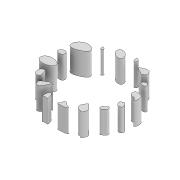
# Autodesk Inventor part: simple_ring3
Saved by Autodesk Inventor 2021 (Build 250183000, 183)
## iProperties
Created: 2022-04-12
Part Number: simple_ring3
Material: Generic
Document SubType Name: Modeling
Designer: Derm
Density: 1 g/cm^3
Appearance: Default
Author: Derm
Autodesk Inventor part; units mm, degrees
ref_plane "YZ Plane" through (0, 0, 0) normal (1, 0, 0) x (0, 1, 0)
ref_plane "XZ Plane" through (0, 0, 0) normal (0, 1, 0) x (-1, 0, 0)
ref_plane "XY Plane" through (0, 0, 0) normal (0, 0, 1) x (1, 0, 0)
sketch "Sketch1" plane through (0, 0, 0) normal (0, 1, 0) x (-1, 0, 0)
  line L0 (0, 0) -> (10000, 0)
  line L1 (0, 0) -> (9807.8528, -1950.9032) construction
  line L2 (-4839.2703, 7607.7402) -> (-4527.6462, 8434.2216) construction
  line L3 (-4527.6462, 8434.2216) -> (-5367.6765, 9477.4851) construction
  line L4 (-5367.6765, 9477.4851) -> (-6194.1579, 8840.6879) construction
  line L5 (-6194.1579, 8840.6879) -> (-6194.1579, 9938.1469) construction
  line L6 (-6194.1579, 9938.1469) -> (-6979.9927, 8718.748) construction
  line L7 (-6979.9927, 8718.748) -> (-7074.8348, 7865.1688) construction
  line L8 (-7074.8348, 7865.1688) -> (-6248.3534, 7350.3115) construction
  line L9 (-6248.3534, 7350.3115) -> (-5462.5186, 6158.0104) construction
  line L10 (-5462.5186, 6158.0104) -> (-5282.6353, 7062.3446) construction
  line L11 (-5282.6353, 7062.3446) -> (-4839.2703, 7607.7402) construction
  spline S0 degree 4 poles (-4839.2703, 7607.7402) (-4527.6462, 8434.2216) (-5367.6765, 9477.4851) (-6194.1579, 8840.6879) (-6194.1579, 9938.1469) (-6979.9927, 8718.748) (-7074.8348, 7865.1688) (-6248.3534, 7350.3115) (-5462.5186, 6158.0104) (-5282.6353, 7062.3446) (-4839.2703, 7607.7402) knots 1 1 1 1 1 2 3 4 5 6 7 8 8 8 8 8
  line L12 (-8998.7753, -2526.8192) -> (-8511.0158, -1632.5933) construction
  line L13 (-8511.0158, -1632.5933) -> (-9486.5348, -711.2697) construction
  line L14 (-9486.5348, -711.2697) -> (-10258.8207, -1293.8714) construction
  line L15 (-10258.8207, -1293.8714) -> (-10773.678, -386.0967) construction
  line L16 (-10773.678, -386.0967) -> (-10673.6173, 116.9424) construction
  line L17 (-10673.6173, 116.9424) -> (-11274.9864, -657.0742) construction
  line L18 (-11274.9864, -657.0742) -> (-11274.9864, -1402.2624) construction
  line L19 (-11274.9864, -1402.2624) -> (-10976.9111, -2526.8192) construction
  line L20 (-10976.9111, -2526.8192) -> (-9807.8528, -2526.8192) construction
  line L21 (-9807.8528, -2526.8192) -> (-8998.7753, -2526.8192) construction
  spline S1 degree 4 poles (-8998.7753, -2526.8192) (-8511.0158, -1632.5933) (-9486.5348, -711.2697) (-10258.8207, -1293.8714) (-10773.678, -386.0967) (-10673.6173, 116.9424) (-11274.9864, -657.0742) (-11274.9864, -1402.2624) (-10976.9111, -2526.8192) (-9807.8528, -2526.8192) (-8998.7753, -2526.8192) knots 1 1 1 1 1 2 3 4 5 6 7 8 8 8 8 8
  line L22 (-3999.2401, -8583.1668) -> (-3999.2401, -7924.4901) construction
  line L23 (-3999.2401, -7924.4901) -> (-5354.1276, -7924.4901) construction
  line L24 (-5354.1276, -7924.4901) -> (-5354.1276, -7119.8881) construction
  line L25 (-5354.1276, -7119.8881) -> (-6085.7669, -7445.0612) construction
  line L26 (-6085.7669, -7445.0612) -> (-7020.6393, -7924.4901) construction
  line L27 (-7020.6393, -7924.4901) -> (-6397.391, -8420.5803) construction
  line L28 (-6397.391, -8420.5803) -> (-6500.0442, -8936.6526) construction
  line L29 (-6500.0442, -8936.6526) -> (-5476.0675, -9436.746) construction
  line L30 (-5476.0675, -9436.746) -> (-4500.5485, -8799.9488) construction
  line L31 (-4500.5485, -8799.9488) -> (-3999.2401, -8583.1668) construction
  spline S2 degree 4 poles (-3999.2401, -8583.1668) (-3999.2401, -7924.4901) (-5354.1276, -7924.4901) (-5354.1276, -7119.8881) (-6085.7669, -7445.0612) (-7020.6393, -7924.4901) (-6397.391, -8420.5803) (-6500.0442, -8936.6526) (-5476.0675, -9436.746) (-4500.5485, -8799.9488) (-3999.2401, -8583.1668) knots 1 1 1 1 1 2 3 4 5 6 7 8 8 8 8 8
  line L32 (8005.0639, 4532.1453) -> (7747.6353, 4911.5139) construction
  line L33 (7747.6353, 4911.5139) -> (7747.6353, 5697.3487) construction
  line L34 (7747.6353, 5697.3487) -> (7232.778, 6103.815) construction
  line L35 (7232.778, 6103.815) -> (7476.6578, 6605.1234) construction
  line L36 (7476.6578, 6605.1234) -> (8314.6961, 7025.1386) construction
  line L37 (8314.6961, 7025.1386) -> (9075.4251, 6225.7549) construction
  line L38 (9075.4251, 6225.7549) -> (9075.4251, 5656.7021) construction
  line L39 (9075.4251, 5656.7021) -> (9075.4251, 5074.1004) construction
  line L40 (9075.4251, 5074.1004) -> (8723.1543, 4626.9875) construction
  line L41 (8723.1543, 4626.9875) -> (8005.0639, 4532.1453) construction
  spline S3 degree 4 poles (8005.0639, 4532.1453) (7747.6353, 4911.5139) (7747.6353, 5697.3487) (7232.778, 6103.815) (7476.6578, 6605.1234) (8314.6961, 7025.1386) (9075.4251, 6225.7549) (9075.4251, 5656.7021) (9075.4251, 5074.1004) (8723.1543, 4626.9875) (8005.0639, 4532.1453) knots 1 1 1 1 1 2 3 4 5 6 7 8 8 8 8 8
  line L42 (2531.318, 10954.3126) -> (2531.318, 10073.6357) construction
  line L43 (2531.318, 10073.6357) -> (2436.4759, 8786.4924) construction
  line L44 (2436.4759, 8786.4924) -> (1460.9569, 9260.7031) construction
  line L45 (1460.9569, 9260.7031) -> (1460.9569, 9965.2447) construction
  line L46 (1460.9569, 9965.2447) -> (878.3552, 10845.9216) construction
  line L47 (878.3552, 10845.9216) -> (1474.5057, 10954.3126) construction
  line L48 (1474.5057, 10954.3126) -> (1826.7765, 10629.1396) construction
  line L49 (1826.7765, 10629.1396) -> (2531.318, 10954.3126) construction
  spline S4 degree 4 poles (2531.318, 10954.3126) (2531.318, 10073.6357) (2436.4759, 8786.4924) (1460.9569, 9260.7031) (1460.9569, 9965.2447) (878.3552, 10845.9216) (1474.5057, 10954.3126) (1826.7765, 10629.1396) (2531.318, 10954.3126) knots 1 1 1 1 1 2 3 4 5 6 6 6 6 6
  line L50 (-1386.8766, -10501.0873) -> (-1386.8766, -9685.4792) construction
  line L51 (-1386.8766, -9685.4792) -> (-1777.6107, -8936.6526) construction
  line L52 (-1777.6107, -8936.6526) -> (-2212.585, -9252.99) construction
  line L53 (-2212.585, -9252.99) -> (-2732.1854, -10059.2666) construction
  line L54 (-2732.1854, -10059.2666) -> (-1386.8766, -10501.0873) construction
  spline S5 degree 4 poles (-1386.8766, -10501.0873) (-1386.8766, -9685.4792) (-1777.6107, -8936.6526) (-2212.585, -9252.99) (-2732.1854, -10059.2666) (-1386.8766, -10501.0873) knots 1 1 1 1 1 2 3 3 3 3 3
  line L55 (6238.4805, 8506.3447) -> (6238.4805, 9153.4105) construction
  line L56 (6238.4805, 9153.4105) -> (5103.2076, 9260.7031) construction
  line L57 (5103.2076, 9260.7031) -> (4785.0565, 8291.9584) construction
  line L58 (4785.0565, 8291.9584) -> (4138.6539, 7471.7517) construction
  line L59 (4138.6539, 7471.7517) -> (4082.6646, 6625.4467) construction
  line L60 (4082.6646, 6625.4467) -> (3686.2076, 7215.1404) construction
  line L61 (3686.2076, 7215.1404) -> (3704.1882, 6625.4467) construction
  line L62 (3704.1882, 6625.4467) -> (4389.4164, 6591.3632) construction
  line L63 (4389.4164, 6591.3632) -> (5484.1105, 7264.4944) construction
  line L64 (5484.1105, 7264.4944) -> (6565.6616, 7865.1688) construction
  line L65 (6565.6616, 7865.1688) -> (6486.4621, 8580.8185) construction
  line L66 (6486.4621, 8580.8185) -> (6238.4805, 8506.3447) construction
  spline S6 degree 4 poles (6238.4805, 8506.3447) (6238.4805, 9153.4105) (5103.2076, 9260.7031) (4785.0565, 8291.9584) (4138.6539, 7471.7517) (4082.6646, 6625.4467) (3686.2076, 7215.1404) (3704.1882, 6625.4467) (4389.4164, 6591.3632) (5484.1105, 7264.4944) (6565.6616, 7865.1688) (6486.4621, 8580.8185) (6238.4805, 8506.3447) knots 1 1 1 1 1 2 3 4 5 6 7 8 9 10 10 10 10 10
  line L67 (-10258.8207, 1567.5332) -> (-9055.5617, 1733.5188) construction
  line L68 (-9055.5617, 1733.5188) -> (-9243.9564, 2541.5805) construction
  line L69 (-9243.9564, 2541.5805) -> (-9927.0456, 3577.9918) construction
  line L70 (-9927.0456, 3577.9918) -> (-11274.9864, 2806.0191) construction
  line L71 (-11274.9864, 2806.0191) -> (-10773.678, 2051.934) construction
  line L72 (-10773.678, 2051.934) -> (-10260.231, 1574.5822) construction
  line L73 (-10260.231, 1574.5822) -> (-10258.8207, 1567.5332) construction
  spline S7 degree 4 poles (-10258.8207, 1567.5332) (-9055.5617, 1733.5188) (-9243.9564, 2541.5805) (-9927.0456, 3577.9918) (-11274.9864, 2806.0191) (-10773.678, 2051.934) (-10260.231, 1574.5822) (-10258.8207, 1567.5332) knots 1 1 1 1 1 2 3 4 5 5 5 5 5
  spline S8 degree 5 poles (10355.9276, -5999.0073) (10649.458, -5515.5439) (10856.7295, -4614.8284) (10271.0092, -3456.1239) (7691.5575, -4638.4703) (5394.0876, -5813.0681) (7385.4507, -7575.4016) (9200.8833, -7264.6674) (10042.4191, -6515.3759) (10355.9276, -5999.0073) knots 0 0 0 0 0 0 0.232539 0.387238 0.587238 0.751634 1 1 1 1 1 1
  spline S9 degree 5 poles (-8449.8988, -5999.0073) (-8270.7148, -6000.0586) (-7963.0266, -5904.0433) (-7561.5505, -5517.4649) (-7605.652, -4794.9789) (-9417.8904, -4758.8853) (-9251.3636, -5509.4109) (-8916.4189, -5900.0705) (-8627.4473, -5997.9656) (-8449.8988, -5999.0073) knots 0 0 0 0 0 0 0.240305 0.401508 0.601508 0.761889 1 1 1 1 1 1
  spline S10 degree 5 poles (5670.844, -8491.9009) (5725.3959, -8473.6627) (5772.4807, -8372.3907) (5720.5336, -8001.1186) (5621.7836, -7284.8578) (4776.674, -8187.0217) (5151.6925, -8266.201) (5475.6182, -8470.1795) (5616.2591, -8510.1502) (5670.844, -8491.9009) knots 0 0 0 0 0 0 0.233443 0.396735 0.596735 0.766415 1 1 1 1 1 1
  spline S11 degree 4 poles (-1331.2246, 10276.4436) (-1776.1213, 10274.596) (-1354.5409, 10035.4129) (-1920.062, 8549.694) (-2722.1204, 9717.3679) (-2994.8101, 9792.5836) (-4164.2812, 10122.318) (-3478.0526, 10483.9401) (-2645.3487, 10689.2135) (-2009.8769, 10553.1497) (-892.0195, 10824.7194) (-1331.2246, 10276.4436) knots 0 0 0 0 0 0.204034 0.298984 0.396709 0.488101 0.578803 0.671721 0.767842 1 1 1 1 1
  spline S12 degree 5 poles (-8314.6961, 5198.8536) (-8242.1823, 5190.4681) (-8056.5984, 5192.6235) (-7598.1036, 5507.3252) (-8208.0894, 6713.9442) (-8579.4288, 5864.8564) (-9381.2159, 5468.2573) (-9461.0905, 5461.8072) (-9056.5369, 3823.7538) (-8432.2819, 5146.5276) (-8432.9842, 5227.5203) (-8371.4871, 5205.4208) (-8314.6961, 5198.8536) knots 0 0 0 0 0 0 0.152178 0.260368 0.391673 0.529991 0.667025 0.789008 0.880818 1 1 1 1 1 1
  spline S13 degree 5 poles (9351.7652, -2315.8498) (9220.3136, -2158.6875) (9099.5439, -1813.759) (9221.3135, -1236.3535) (9612.8935, -1051.4256) (11546.3276, -1176.3365) (10756.1187, -2560.2421) (9894.8855, -2703.1112) (9505.8474, -2500.069) (9351.7652, -2315.8498) knots 0 0 0 0 0 0 0.220201 0.378255 0.578255 0.74189 1 1 1 1 1 1
  spline S14 degree 5 poles (10997.4506, 1076.3286) (11552.3966, 1379.5959) (12144.3228, 2232.979) (11575.9513, 3922.6337) (7479.0356, 3224.9367) (6927.4968, 1623.9927) (9041.9335, 597.9662) (10403.7811, 751.8996) (10997.4506, 1076.3286) knots 0 0 0 0 0 0 0.289886 0.489886 0.689886 1 1 1 1 1 1
  spline S15 degree 5 poles (2490.9307, -10280.177) (2856.7217, -10168.5286) (3288.6877, -9660.8702) (3065.982, -8299.8946) (81.9324, -7231.6907) (3.765, -9055.7868) (1235.5712, -10238.4669) (2095.9782, -10400.7261) (2490.9307, -10280.177) knots 0 0 0 0 0 0 0.2885 0.4885 0.6885 1 1 1 1 1 1
  point P0 (9807.8528, 1950.9032)
  point P1 (8314.6961, 5555.7023)
  point P2 (5555.7023, 8314.6961)
  point P3 (1950.9032, 9807.8528)
  point P4 (-1950.9032, 9807.8528)
  point P5 (-5555.7023, 8314.6961)
  point P6 (-8314.6961, 5555.7023)
  point P7 (-9807.8528, 1950.9032)
  point P8 (-9807.8528, -1950.9032)
  point P9 (-8314.6961, -5555.7023)
  point P10 (-5555.7023, -8314.6961)
  point P11 (-1950.9032, -9807.8528)
  point P12 (1950.9032, -9807.8528)
  point P13 (5555.7023, -8314.6961)
  point P14 (8314.6961, -5555.7023)
  point P15 (9154.6321, -1820.9695)
  point P16 (7876.3496, -4624.774)
  point P17 (6486.4621, -5999.0073)
  point P18 (7895.6769, -7119.8881)
  point P19 (-7901.8948, -5054.8661)
  point P20 (-9055.5617, -5044.1211)
  point P21 (-9055.5617, -5646.4814)
  point P22 (5484.1105, -7684.7756)
  point P23 (5058.3585, -8076.8552)
  point P24 (5325.8324, -8376.6104)
  point P25 (-1582.2435, 10159.7078)
  point P26 (-1658.8525, 9612.9733)
  point P27 (-2091.8966, 9153.4094)
  point P28 (-2673.2449, 9572.4274)
  point P29 (-3191.3093, 9848.2369)
  point P30 (-3812.2129, 10165.6403)
  point P31 (-3568.9955, 10405.583)
  point P32 (-2916.4851, 10591.3455)
  point P33 (-2212.585, 10629.1396)
  point P34 (-1326.4343, 10629.1399)
  point P35 (-8123.5987, 6181.6268)
  point P36 (-8631.0724, 5989.99)
  point P37 (-9243.9564, 5519.5703)
  point P38 (-9328.7655, 5074.1004)
  point P39 (-8852.8938, 4579.5664)
  point P40 (-8403.521, 5198.8536)
  point P41 (9706.617, -1171.9315)
  point P42 (10863.6676, -1484.1264)
  point P43 (10363.5607, -2458.2081)
  point P44 (8220.7484, 2806.0191)
  point P45 (7895.6769, 1574.5822)
  point P46 (783.0728, -8076.8552)
  point P47 (581.9894, -9248.6798)
  dimension "d1" = 11.25
  dimension "d4" = 360
  constraints: 11 vertical, 4 end point, 4 horizontal, 2 coincident, 1 point on line, 83 other
  measures "d1" angle of L1 L0
extrude "Extrusion2" add sketch "Sketch1" along normal blind 3000
mirror "Mirror1" about plane through (-1646.2264, 0, -8816.2084) normal (0, -1, 0) of "Extrusion2"
body "Solid2"
